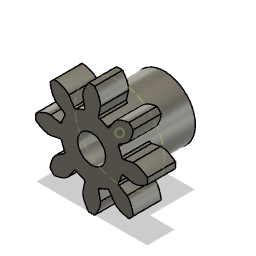
gear1245 v13 (Autodesk Fusion 360 design; units mm, degrees)
description: middle size
description: Spur Gear; Module: 2.0; Num Teeth: 8; Pressure Angle: 20.0; Backlash: 0.00 mm
Autodesk Fusion 360 part; units mm, degrees
sketch "草图1" plane through (0, 0, 0) normal (0, 0, 1) x (1, 0, 0) in component "Spur Gear (8 teeth)"
  circle A0 centre (0, 0) radius 5.5492
  circle A1 centre (0, 0) radius 2.5
extrude "拉伸1" add sketch "草图1" along normal blind 5 and the other way blind 8 in component "Spur Gear (8 teeth)"
sketch "草图2" plane through (0, 0, 0) normal (0, 0, 1) x (1, 0, 0) in component "Spur Gear (8 teeth)"
  spline S0 degree 5 poles (7.3504, -1.5763) (7.3577, -1.5779) (7.3723, -1.5807) (7.3943, -1.5841) (7.4239, -1.5871) (7.4612, -1.5888) (7.4987, -1.5889) (7.5364, -1.588) (7.5741, -1.5866) (7.6119, -1.5849) (7.6498, -1.5827) (7.6877, -1.5801) (7.7257, -1.5767) (7.7638, -1.5726) (7.802, -1.5677) (7.8402, -1.562) (7.8785, -1.5558) (7.9168, -1.549) (7.9551, -1.5418) (7.9935, -1.5341) (8.0319, -1.526) (8.0703, -1.5174) (8.1087, -1.5082) (8.1471, -1.4986) (8.1856, -1.4885) (8.224, -1.4779) (8.2624, -1.4668) (8.3009, -1.4553) (8.3393, -1.4434) (8.3778, -1.4311) (8.4162, -1.4183) (8.4546, -1.4051) (8.4929, -1.3915) (8.5313, -1.3774) (8.5696, -1.363) (8.608, -1.3481) (8.6462, -1.3328) (8.6845, -1.3172) (8.7227, -1.3011) (8.7609, -1.2847) (8.799, -1.2679) (8.8371, -1.2506) (8.8752, -1.2331) (8.9132, -1.2151) (8.9512, -1.1967) (8.9891, -1.178) (9.0269, -1.1589) (9.0647, -1.1395) (9.1025, -1.1197) (9.1401, -1.0995) (9.1778, -1.079) (9.2153, -1.0581) (9.2528, -1.0368) (9.2902, -1.0152) (9.3276, -0.9933) (9.3648, -0.971) (9.402, -0.9484) (9.4392, -0.9254) (9.4762, -0.9021) (9.5132, -0.8784) (9.55, -0.8544) (9.5868, -0.8301) (9.6235, -0.8055) (9.6602, -0.7805) (9.6967, -0.7552) (9.7331, -0.7295) (9.7695, -0.7036) (9.8057, -0.6773) (9.8418, -0.6507) (9.8779, -0.6238) (9.9138, -0.5965) (9.9425, -0.5745) (9.9639, -0.5578) (9.9782, -0.5466) (9.9854, -0.541) knots 0 0 0 0 0 0 0.01428571 0.02857143 0.04285714 0.05714286 0.07142857 0.08571429 0.1 0.11428571 0.12857143 0.14285714 0.15714286 0.17142857 0.18571429 0.2 0.21428571 0.22857143 0.24285714 0.25714286 0.27142857 0.28571429 0.3 0.31428571 0.32857143 0.34285714 0.35714286 0.37142857 0.38571429 0.4 0.41428571 0.42857143 0.44285714 0.45714286 0.47142857 0.48571429 0.5 0.51428571 0.52857143 0.54285714 0.55714286 0.57142857 0.58571429 0.6 0.61428571 0.62857143 0.64285714 0.65714286 0.67142857 0.68571429 0.7 0.71428571 0.72857143 0.74285714 0.75714286 0.77142857 0.78571429 0.8 0.81428571 0.82857143 0.84285714 0.85714286 0.87142857 0.88571429 0.9 0.91428571 0.92857143 0.94285714 0.95714286 0.97142857 0.98571429 1 1 1 1 1 1
  spline S1 degree 5 poles (7.3504, 1.5763) (7.3577, 1.5779) (7.3723, 1.5807) (7.3943, 1.5841) (7.4239, 1.5871) (7.4612, 1.5888) (7.4987, 1.5889) (7.5364, 1.588) (7.5741, 1.5866) (7.6119, 1.5849) (7.6498, 1.5827) (7.6877, 1.5801) (7.7257, 1.5767) (7.7638, 1.5726) (7.802, 1.5677) (7.8402, 1.562) (7.8785, 1.5558) (7.9168, 1.549) (7.9551, 1.5418) (7.9935, 1.5341) (8.0319, 1.526) (8.0703, 1.5174) (8.1087, 1.5082) (8.1471, 1.4986) (8.1856, 1.4885) (8.224, 1.4779) (8.2624, 1.4668) (8.3009, 1.4553) (8.3393, 1.4434) (8.3778, 1.4311) (8.4162, 1.4183) (8.4546, 1.4051) (8.4929, 1.3915) (8.5313, 1.3774) (8.5696, 1.363) (8.608, 1.3481) (8.6462, 1.3328) (8.6845, 1.3172) (8.7227, 1.3011) (8.7609, 1.2847) (8.799, 1.2679) (8.8371, 1.2506) (8.8752, 1.2331) (8.9132, 1.2151) (8.9512, 1.1967) (8.9891, 1.178) (9.0269, 1.1589) (9.0647, 1.1395) (9.1025, 1.1197) (9.1401, 1.0995) (9.1778, 1.079) (9.2153, 1.0581) (9.2528, 1.0368) (9.2902, 1.0152) (9.3276, 0.9933) (9.3648, 0.971) (9.402, 0.9484) (9.4392, 0.9254) (9.4762, 0.9021) (9.5132, 0.8784) (9.55, 0.8544) (9.5868, 0.8301) (9.6235, 0.8055) (9.6602, 0.7805) (9.6967, 0.7552) (9.7331, 0.7295) (9.7695, 0.7036) (9.8057, 0.6773) (9.8418, 0.6507) (9.8779, 0.6238) (9.9138, 0.5965) (9.9425, 0.5745) (9.9639, 0.5578) (9.9782, 0.5466) (9.9854, 0.541) knots 0 0 0 0 0 0 0.01428571 0.02857143 0.04285714 0.05714286 0.07142857 0.08571429 0.1 0.11428571 0.12857143 0.14285714 0.15714286 0.17142857 0.18571429 0.2 0.21428571 0.22857143 0.24285714 0.25714286 0.27142857 0.28571429 0.3 0.31428571 0.32857143 0.34285714 0.35714286 0.37142857 0.38571429 0.4 0.41428571 0.42857143 0.44285714 0.45714286 0.47142857 0.48571429 0.5 0.51428571 0.52857143 0.54285714 0.55714286 0.57142857 0.58571429 0.6 0.61428571 0.62857143 0.64285714 0.65714286 0.67142857 0.68571429 0.7 0.71428571 0.72857143 0.74285714 0.75714286 0.77142857 0.78571429 0.8 0.81428571 0.82857143 0.84285714 0.85714286 0.87142857 0.88571429 0.9 0.91428571 0.92857143 0.94285714 0.95714286 0.97142857 0.98571429 1 1 1 1 1 1
  arc A0 (9.9854, -0.541) -> (9.9854, 0.541) centre (0, 0) ccw
  line L0 (5.4161, -1.1636) -> (7.3504, -1.5763)
  line L1 (5.4161, 1.1636) -> (7.3504, 1.5763)
  line L2 (5.4161, -1.1636) -> (5.4161, 1.1636)
  point P0 (7.5292, -1.5881)
  point P1 (7.7124, -1.5778)
  point P2 (7.8984, -1.5522)
  point P3 (8.0864, -1.5135)
  point P4 (8.2759, -1.4628)
  point P5 (8.4663, -1.4008)
  point P6 (8.6575, -1.3282)
  point P7 (8.8489, -1.2451)
  point P8 (9.0403, -1.152)
  point P9 (9.2313, -1.049)
  point P10 (9.4216, -0.9362)
  point P11 (9.611, -0.8139)
  point P12 (9.799, -0.6821)
  point P13 (7.5292, 1.5881)
  point P14 (7.7124, 1.5778)
  point P15 (7.8984, 1.5522)
  point P16 (8.0864, 1.5135)
  point P17 (8.2759, 1.4628)
  point P18 (8.4663, 1.4008)
  point P19 (8.6575, 1.3282)
  point P20 (8.8489, 1.2451)
  point P21 (9.0403, 1.152)
  point P22 (9.2313, 1.049)
  point P23 (9.4216, 0.9362)
  point P24 (9.611, 0.8139)
  point P25 (9.799, 0.6821)
extrude "拉伸2" add sketch "草图2" along normal blind 5 in component "Spur Gear (8 teeth)"
fillet "圆角1" radius 0.3 2 edges at (5.4254, -1.1656, 2.5) (5.4254, 1.1656, 2.5) in component "Spur Gear (8 teeth)"
pattern_circular "C-阵列1" count 8 over 360 about axis through (0, 0, -8) along (0, 0, 1) of "拉伸2", "圆角1" in component "Spur Gear (8 teeth)"
sketch "草图3" plane through (0, 0, 0) normal (0, 0, 1) x (1, 0, 0) in component "Spur Gear (8 teeth)"
  circle A0 centre (0, 0) radius 8 construction
component "Spur Gear (8 teeth)" placed x (1, 0, 0) y (0, 1, 0) z (0, 0, 1) at (0, 0, 0)
